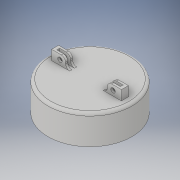
# Autodesk Inventor part: Base with 9V Batt
Saved by Autodesk Inventor 2018.3 (Build 223284000, 284)
## iProperties
Company: UNH Makerspace
Created: 2019-07-26
Part Number: Base with 9V Batt
Material: Generic
Document SubType Name: Modeling
Designer: Electro707
Density: 1 g/cm^3
Appearance: Default
Engineer: Jamal Bouajjaj
Description: The base for the main PCB
Mass: 35.02 g
Surface Area: 144.569 cm^2
Volume: 35.02 cm^3
Author: Electro707
Title: Dual Construction Tree - Base
Revision Number: N/A
Autodesk Inventor part; units mm, degrees
ref_plane "Work Plane2" through (0, 0, 32.5) normal (0, 0, 1) x (1, 0, 0)
ref_plane "YZ Plane" through (0, 0, 0) normal (1, 0, 0) x (0, 1, 0)
sketch "Sketch1" plane through (0, 0, 0) normal (0, 0, 1) x (1, 0, 0)
  line L0 (25, 7) -> (-25, 7)
  line L1 (-25, 7) -> (-25, 0)
  line L2 (-25, 0) -> (25, 0)
  line L3 (25, 0) -> (25, 7)
  circle A0 centre (-19, 3.5) radius 1.6
  circle A1 centre (19, 3.5) radius 1.6
  line L4 (19, 3.5) -> (-19, 3.5) construction
  line L5 (19, 3.5) -> (25, 7) construction
  line L6 (19, 3.5) -> (25, 0) construction
  line L7 (-19, 3.5) -> (-25, 7) construction
  line L8 (-19, 3.5) -> (-25, 0) construction
  line L9 (0, 0) -> (-19, 3.5) construction
  line L10 (0, 0) -> (19, 3.5) construction
  dimension "d0" = 3.2
  dimension "d1" = 38
  dimension "d2" = 7
  dimension "d3" = 50
  constraints: 22 end point, 4 equal length, 2 centre point, 2 horizontal, 2 parallel, 1 equal radius, 1 midpoint, 1 perpendicular
  measures "d0" diameter of A1
  measures "d1" distance of L4.start L4.end
  measures "d2" distance of L0.end L1.end
  measures "d3" distance of L0.start L0.end
extrude "Extrusion1" add sketch "Sketch1" along normal blind 5
sketch "Sketch2" plane through (-25, 7, 0) normal (0, 1, 0) x (1, 0, 0)
  line L0 (2.25, -3.5) -> (10, -3.5)
  line L1 (47.75, -3.5) -> (47.75, -1.5)
  line L2 (47.75, -1.5) -> (40, -1.5)
  line L3 (2.25, -1.5) -> (2.25, -3.5)
  line L4 (50, -5) -> (0, -5) construction
  line L5 (0, -5) -> (2.25, -3.5) construction
  line L6 (50, 0) -> (0, 0) construction
  line L7 (2.25, -1.5) -> (0, 0) construction
  line L8 (50, 0) -> (50, -5) construction
  line L9 (47.75, -3.5) -> (50, -5) construction
  line L10 (40, -3.5) -> (40, -5)
  line L11 (40, -5) -> (10, -5)
  line L12 (10, -5) -> (10, -3.5)
  line L13 (10, -1.5) -> (10, 0)
  line L14 (10, 0) -> (40, 0)
  line L15 (40, 0) -> (40, -1.5)
  line L16 (40, -3.5) -> (47.75, -3.5)
  line L17 (40, -1.5) -> (10, -1.5) construction
  line L18 (10, -3.5) -> (40, -3.5) construction
  line L19 (10, -1.5) -> (2.25, -1.5)
  line L20 (47.75, -3.5) -> (40, -5) construction
  line L21 (40, 0) -> (47.75, -1.5) construction
  line L22 (10, -5) -> (2.25, -3.5) construction
  line L23 (2.25, -1.5) -> (10, 0) construction
  point P0 (25, 0)
  dimension "d6" = 45.5
  dimension "d7" = 2
  dimension "d13" = 30
  constraints: 42 end point, 10 parallel, 9 perpendicular, 6 point on line, 5 equal length, 3 horizontal, 2 collinear
  measures "d6" distance of L1.end L3.start
  measures "d7" distance of L3.start L0.start
  measures "d13" distance of L10.end L11.end
extrude "Extrusion2" cut sketch "Sketch2" against normal up to next
sketch "Sketch3" plane through (-25, 0, 0) normal (0, -1, 0) x (1, 0, 0)
  circle A0 centre (25, 2.5) radius 30
  line L0 (0, 5) -> (50, 5) construction
  line L1 (0, 5) -> (25, 2.5) construction
  line L2 (0, 0) -> (50, 0) construction
  line L3 (25, 2.5) -> (0, 0) construction
  line L4 (25, 2.5) -> (50, 5) construction
  point P0 (25, 0)
  dimension "d10" = 60
  constraints: 6 end point, 2 equal length, 1 centre point
  measures "d10" diameter of A0
extrude "Extrusion3" add sketch "Sketch3" along normal blind 21
ref_plane "Work Plane1" through (0, 0, -27.5) normal (0, 0, 1) x (1, 0, 0)
sketch "Sketch5" plane through (0, 0, -27.5) normal (0, 0, 1) x (1, 0, 0)
  line L0 (14, -1.5) -> (-14, -1.5)
  line L1 (-14, -1.5) -> (-14, -19.5)
  line L2 (-14, -19.5) -> (14, -19.5)
  line L3 (14, -19.5) -> (14, -1.5)
  line L4 (-30, -21) -> (30, -21) construction
  line L5 (30, 0) -> (-30, 0) construction
  line L6 (30, 0) -> (-30, 0) construction
  line L7 (30, 0) -> (14, -1.5) construction
  line L8 (-14, -1.5) -> (-30, 0) construction
  line L9 (-30, -21) -> (30, -21) construction
  line L10 (-30, -21) -> (-14, -19.5) construction
  point P0 (0, 0)
  dimension "d16" = 18
  dimension "d17" = 28
  constraints: 14 end point, 2 equal length, 2 parallel, 1 horizontal, 1 perpendicular
  measures "d16" distance of L2.end L0.start
  measures "d17" distance of L0.start L0.end
extrude "Extrusion4" cut sketch "Sketch5" along normal blind 50
fillet "Fillet1" radius 3 8 edges at (15, 7, 0.75) (15, 7, 4.25) (15, 0, 4.25) (15, 0, 0.75) (-15, 0, 0.75) (-15, 7, 0.75) (-15, 7, 4.25) (-15, 0, 4.25)
fillet "Fillet2" radius 2 1 edges at (-30, 0, 2.5)
sketch "Sketch7" plane through (0, 0, 32.5) normal (0, 0, 1) x (1, 0, 0)
  spline S0 degree 3 poles (3.6755, -17.8887) (1.3417, -19.2361) (-1.5336, -19.2361) (-3.8674, -17.8887) knots 0 0 0 0 1 1 1 1
  line L0 (3.6755, -17.8887) -> (1.3417, -19.2361) construction
  line L1 (1.3417, -19.2361) -> (-1.5336, -19.2361) construction
  line L2 (-1.5336, -19.2361) -> (-3.8674, -17.8887) construction
  spline S1 degree 3 poles (-3.8674, -17.8887) (-6.2011, -16.5413) (-7.6388, -14.0512) (-7.6388, -11.3564) knots 0 0 0 0 1 1 1 1
  line L3 (-3.8674, -17.8887) -> (-6.2011, -16.5413) construction
  line L4 (-6.2011, -16.5413) -> (-7.6388, -14.0512) construction
  line L5 (-7.6388, -14.0512) -> (-7.6388, -11.3564) construction
  spline S2 degree 3 poles (-7.6388, -11.3564) (-7.6388, -8.6616) (-6.2011, -6.1715) (-3.8674, -4.8241) knots 0 0 0 0 1 1 1 1
  line L6 (-7.6388, -11.3564) -> (-7.6388, -8.6616) construction
  line L7 (-7.6388, -8.6616) -> (-6.2011, -6.1715) construction
  line L8 (-6.2011, -6.1715) -> (-3.8674, -4.8241) construction
  spline S3 degree 3 poles (-3.8674, -4.8241) (-1.5336, -3.4767) (1.3417, -3.4767) (3.6755, -4.8241) knots 0 0 0 0 1 1 1 1
  line L9 (-3.8674, -4.8241) -> (-1.5336, -3.4767) construction
  line L10 (-1.5336, -3.4767) -> (1.3417, -3.4767) construction
  line L11 (1.3417, -3.4767) -> (3.6755, -4.8241) construction
  spline S4 degree 3 poles (3.6755, -4.8241) (6.0092, -6.1715) (7.4469, -8.6616) (7.4469, -11.3564) knots 0 0 0 0 1 1 1 1
  line L12 (3.6755, -4.8241) -> (6.0092, -6.1715) construction
  line L13 (6.0092, -6.1715) -> (7.4469, -8.6616) construction
  line L14 (7.4469, -8.6616) -> (7.4469, -11.3564) construction
  spline S5 degree 3 poles (7.4469, -11.3564) (7.4469, -14.0512) (6.0092, -16.5413) (3.6755, -17.8887) knots 0 0 0 0 1 1 1 1
  line L15 (7.4469, -11.3564) -> (7.4469, -14.0512) construction
  line L16 (7.4469, -14.0512) -> (6.0092, -16.5413) construction
  line L17 (6.0092, -16.5413) -> (3.6755, -17.8887) construction
  spline S6 degree 3 poles (-0.623, -14.5187) (-0.623, -14.5201) (-0.623, -15.9241) (-2.0285, -15.9241) knots 0 0 0 0 1 1 1 1
  line L18 (-0.623, -14.5187) -> (-0.623, -14.5187) construction
  line L19 (-0.623, -14.5187) -> (-0.623, -15.9241) construction
  line L20 (-0.623, -15.9241) -> (-2.0285, -15.9241) construction
  spline S7 degree 3 poles (-2.0285, -15.9241) (-3.4339, -15.9241) (-3.4339, -14.5201) (-3.4339, -14.5187) knots 0 0 0 0 1 1 1 1
  line L21 (-2.0285, -15.9241) -> (-3.4339, -15.9241) construction
  line L22 (-3.4339, -15.9241) -> (-3.4339, -14.5187) construction
  line L23 (-3.4339, -14.5187) -> (-3.4339, -14.5187) construction
  line L24 (-0.623, -5.7345) -> (-0.623, -14.5187)
  spline S8 degree 3 poles (-4.488, -14.5187) (-4.488, -14.5211) (-4.488, -16.9782) (-2.0285, -16.9782) knots 0 0 0 0 1 1 1 1
  line L25 (-4.488, -14.5187) -> (-4.488, -14.5187) construction
  line L26 (-4.488, -14.5187) -> (-4.488, -16.9782) construction
  line L27 (-4.488, -16.9782) -> (-2.0285, -16.9782) construction
  spline S9 degree 3 poles (-2.0285, -16.9782) (0.4311, -16.9782) (0.4311, -14.5211) (0.4311, -14.5187) knots 0 0 0 0 1 1 1 1
  line L28 (-2.0285, -16.9782) -> (0.4311, -16.9782) construction
  line L29 (0.4311, -16.9782) -> (0.4311, -14.5187) construction
  line L30 (0.4311, -14.5187) -> (0.4311, -14.5187) construction
  line L31 (-3.4339, -14.5187) -> (-4.488, -14.5187)
  spline S10 degree 3 poles (1.8366, -14.5187) (1.839, -14.5187) (4.2961, -14.5187) (4.2961, -12.0591) knots 0 0 0 0 1 1 1 1
  line L32 (1.8366, -14.5187) -> (1.8366, -14.5187) construction
  line L33 (1.8366, -14.5187) -> (4.2961, -14.5187) construction
  line L34 (4.2961, -14.5187) -> (4.2961, -12.0591) construction
  spline S11 degree 3 poles (4.2961, -12.0591) (4.2961, -11.0712) (3.8992, -10.4803) (3.4243, -10.1266) knots 0 0 0 0 1 1 1 1
  line L35 (4.2961, -12.0591) -> (4.2961, -11.0712) construction
  line L36 (4.2961, -11.0712) -> (3.8992, -10.4803) construction
  line L37 (3.8992, -10.4803) -> (3.4243, -10.1266) construction
  spline S12 degree 3 poles (3.4243, -10.1266) (3.8992, -9.7729) (4.2961, -9.182) (4.2961, -8.1941) knots 0 0 0 0 1 1 1 1
  line L38 (3.4243, -10.1266) -> (3.8992, -9.7729) construction
  line L39 (3.8992, -9.7729) -> (4.2961, -9.182) construction
  line L40 (4.2961, -9.182) -> (4.2961, -8.1941) construction
  spline S13 degree 3 poles (4.2961, -8.1941) (4.2961, -5.7345) (1.839, -5.7345) (1.8366, -5.7345) knots 0 0 0 0 1 1 1 1
  line L41 (4.2961, -8.1941) -> (4.2961, -5.7345) construction
  line L42 (4.2961, -5.7345) -> (1.8366, -5.7345) construction
  line L43 (1.8366, -5.7345) -> (1.8366, -5.7345) construction
  line L44 (0.4311, -14.5187) -> (1.8366, -14.5187)
  line L45 (1.8366, -5.7345) -> (-0.623, -5.7345)
  spline S14 degree 3 poles (1.8366, -6.7886) (1.838, -6.7886) (3.242, -6.7886) (3.242, -8.1941) knots 0 0 0 0 1 1 1 1
  line L46 (1.8366, -6.7886) -> (1.8366, -6.7886) construction
  line L47 (1.8366, -6.7886) -> (3.242, -6.7886) construction
  line L48 (3.242, -6.7886) -> (3.242, -8.1941) construction
  spline S15 degree 3 poles (3.242, -8.1941) (3.242, -9.5995) (1.838, -9.5995) (1.8366, -9.5995) knots 0 0 0 0 1 1 1 1
  line L49 (3.242, -8.1941) -> (3.242, -9.5995) construction
  line L50 (3.242, -9.5995) -> (1.8366, -9.5995) construction
  line L51 (1.8366, -9.5995) -> (1.8366, -9.5995) construction
  line L52 (0.4311, -6.7886) -> (1.8366, -6.7886)
  line L53 (1.8366, -9.5995) -> (0.4311, -9.5995)
  line L54 (0.4311, -9.5995) -> (0.4311, -6.7886)
  spline S16 degree 3 poles (1.8366, -10.6536) (1.838, -10.6536) (3.242, -10.6536) (3.242, -12.0591) knots 0 0 0 0 1 1 1 1
  line L55 (1.8366, -10.6536) -> (1.8366, -10.6536) construction
  line L56 (1.8366, -10.6536) -> (3.242, -10.6536) construction
  line L57 (3.242, -10.6536) -> (3.242, -12.0591) construction
  spline S17 degree 3 poles (3.242, -12.0591) (3.242, -13.4646) (1.838, -13.4646) (1.8366, -13.4646) knots 0 0 0 0 1 1 1 1
  line L58 (3.242, -12.0591) -> (3.242, -13.4646) construction
  line L59 (3.242, -13.4646) -> (1.8366, -13.4646) construction
  line L60 (1.8366, -13.4646) -> (1.8366, -13.4646) construction
  line L61 (0.4311, -10.6536) -> (1.8366, -10.6536)
  line L62 (1.8366, -13.4646) -> (0.4311, -13.4646)
  line L63 (0.4311, -13.4646) -> (0.4311, -10.6536)
  point P0 (0, 0)
  constraints: 20 end point, 54 other
body "Solid1"
